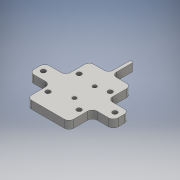
# Autodesk Inventor part: vertical carriage vasi
Saved by Autodesk Inventor 2016 SP1 (Build 200210100, 210)
## iProperties
Created: 2016-03-21
Part Number: vertical carriage vasi
Material: Generic
Document SubType Name: Modeling
Designer: ubik
Density: 1 g/cm^3
Appearance: Default
Author: ubik
Autodesk Inventor part; units mm, degrees
ref_plane "YZ Plane" through (0, 0, 0) normal (1, 0, 0) x (0, 1, 0)
ref_plane "XZ Plane" through (0, 0, 0) normal (0, 1, 0) x (-1, 0, 0)
ref_plane "XY Plane" through (0, 0, 0) normal (0, 0, 1) x (1, 0, 0)
sketch "Sketch1" plane through (0, 0, 0) normal (0, 0, 1) x (1, 0, 0)
  circle A0 centre (-10, 0) radius 1.5
  circle A1 centre (10, 0) radius 1.5
  circle A2 centre (-10, -20) radius 1.5
  circle A3 centre (10, -20) radius 1.5
  line L0 (-15, 10) -> (15, 10)
  line L1 (15, 10) -> (15, -30)
  line L2 (15, -30) -> (-15, -30)
  line L3 (-15, -30) -> (-15, 10)
  point P0 (0, 0)
  dimension "d0" = 3
  dimension "d1" = 3
  dimension "d2" = 20
  dimension "d3" = 10
  dimension "d4" = 3
  dimension "d5" = 3
  dimension "d6" = 20
  dimension "d7" = 20
  dimension "d8" = 20
  dimension "d9" = 10
  dimension "d10" = 30
  dimension "d11" = 15
  dimension "d12" = 40
  dimension "d13" = 10
  constraints: 8 end point, 4 centre point, 2 parallel, 1 horizontal, 1 perpendicular
  measures "d0" diameter of A0
  measures "d1" diameter of A1
  measures "d2" distance of A1.centre A0.centre
  measures "d3" distance of point (0, 0) A0.centre
  measures "d4" diameter of A2
  measures "d5" diameter of A3
  measures "d6" distance of A2.centre A0.centre
  measures "d7" distance of A3.centre A1.centre
  measures "d8" distance of A3.centre A2.centre
  measures "d9" horizontal distance of point (0, 0) A2.centre
  measures "d10" distance of L0.start L0.end
  measures "d11" distance from line of point (0, 0) L3
  measures "d12" distance of L2.end L0.start
  measures "d13" distance from line of point (0, 0) L0
extrude "Extrusion1" add sketch "Sketch1" along normal blind 5
sketch "Sketch2" plane through (0, 0, 5) normal (0, 0, 1) x (1, 0, 0)
  line L0 (0, 15.442053) -> (0, -37.541934) construction
  line L1 (-4, 15.442053) -> (-4, -37.541934) construction
  line L2 (-15, -30) -> (15, -30) construction
  line L3 (15, 10) -> (-15, 10)
  line L4 (15, -30) -> (15, 10)
  line L5 (7, 10) -> (7, -30)
  line L6 (7, 10) -> (15, 10)
  line L7 (7, -30) -> (15, -30)
  line L8 (6.3, 15.442053) -> (6.3, 10) construction
  line L9 (6.3, -30) -> (6.3, -37.541934) construction
  line L10 (-15, 10) -> (-15, -30)
  line L11 (15, -30) -> (15, 10)
  point P0 (0, 0)
  dimension "d16" = 4
  dimension "d96" = 0
  dimension "d97" = 0
  dimension "d141" = 22
  dimension "d152" = 0
  constraints: 16 end point, 4 vertical, 2 perpendicular, 2 point on line, 1 parallel
  measures "d16" distance between parallel lines of L0 L1
  measures "d96" distance between parallel lines of L3 L6
  measures "d97" distance between parallel lines of L2 L7
  measures "d141" distance between parallel lines of L5 L10
  measures "d152" distance between parallel lines of L11 L4
extrude "Extrusion2" add sketch "Sketch2" along normal blind 10
sketch "Sketch4" plane through (0, 0, 15) normal (0, 0, 1) x (1, 0, 0)
  circle A0 centre (10, 0) radius 3.25
  circle A1 centre (10, -20) radius 1.5 projected
  circle A2 centre (10, -20) radius 3.25
  point P0 (0, 0)
  point P1 (8.5, 0)
  point P2 (8.5, -20)
  dimension "d37" = 6.5
  dimension "d38" = 6.5
  constraints: 2 centre point, 2 coincident, 1 horizontal alignment
  measures "d37" diameter of A0
  measures "d38" diameter of A2
extrude "Extrusion3" [suppressed]
sketch "Sketch5" plane through (0, 0, 5) normal (0, 0, 1) x (1, 0, 0)
  line L0 (-4, 15.442053) -> (-4, -37.541934) construction
  line L1 (15, -30) -> (-15, -30)
  line L2 (7, 10) -> (-15, 10)
  line L3 (-3.3, 10) -> (1, 10)
  line L4 (4.5, -30) -> (-3.3, -30)
  line L5 (-3.3, -30) -> (-3.3, 10)
  line L6 (-2, 6) -> (1, 6)
  line L7 (4.5, -26) -> (-2, -26)
  line L8 (-2, -26) -> (-2, 6)
  line L9 (1, 10) -> (1, 6)
  line L10 (4.5, -26) -> (4.5, -30)
  line L11 (7, 10) -> (7, -30)
  point P0 (0, 0)
  point P1 (6.3, 10)
  point P2 (6.3, -30)
  point P3 (15, 10)
  dimension "d111" = 0.7
  dimension "d112" = 4
  dimension "d115" = 4
  dimension "d116" = 1.3
  dimension "d117" = 6
  dimension "d118" = 2.5
  dimension "d139" = 0
  dimension "d140" = 0
  constraints: 16 end point, 4 parallel, 2 horizontal, 2 perpendicular
  measures "d111" distance between parallel lines of L5 L0
  measures "d112" distance between parallel lines of L6 L3
  measures "d115" distance between parallel lines of L4 L7
  measures "d116" distance between parallel lines of L5 L8
  measures "d117" distance between parallel lines of L11 L9
  measures "d118" distance between parallel lines of L11 L10
  measures "d139" distance between parallel lines of L1 L4
  measures "d140" distance between parallel lines of L2 L3
extrude "Extrusion4" add sketch "Sketch5" along normal up to surface (10 mm away) contours L1 L5 L2 L9 L6 L8 L7 L10
sketch "Sketch8" plane through (0, 0, 0) normal (0, 0, -1) x (-1, 0, 0)
  line L0 (27, -15) -> (-27, -15)
  line L1 (-27, -15) -> (-27, -5)
  line L2 (-27, -5) -> (27, -5)
  line L3 (27, -5) -> (27, -15)
  line L4 (15, 10) -> (-15, 10) projected
  line L5 (-15, -30) -> (15, -30) projected
  circle A0 centre (23, -10) radius 1.5
  circle A1 centre (-23, -10) radius 1.5
  point P0 (0, 0)
  dimension "d77" = 10
  dimension "d78" = 40
  dimension "d79" = 15
  dimension "d80" = 3
  dimension "d81" = 3
  dimension "d82" = 46
  dimension "d83" = 54
  dimension "d84" = 23
  dimension "d85" = 27
  constraints: 8 end point, 2 centre point, 2 parallel, 1 horizontal, 1 perpendicular
  measures "d77" distance between parallel lines of L2 L0
  measures "d78" distance between parallel lines of L4 L5
  measures "d79" distance between parallel lines of L5 L0
  measures "d80" diameter of A0
  measures "d81" diameter of A1
  measures "d82" distance of A1.centre A0.centre
  measures "d83" distance of L1.end L2.end
  measures "d84" horizontal distance of point (0, 0) A0.centre
  measures "d85" distance from line of point (0, 0) L3
extrude "Extrusion5" add sketch "Sketch8" against normal up to surface (5 mm away)
sketch "Sketch3" plane through (0, 0, 5) normal (0, 0, 1) x (1, 0, 0)
  circle A0 centre (2, -2) radius 1.25
  circle A1 centre (2, -15) radius 1.25
  line L0 (-15, -30) -> (15, -30) projected
  line L1 (15, 10) -> (-15, 10) projected
  point P0 (0, 0)
  point P1 (7, -30)
  point P2 (6.3, 10)
  dimension "d23" = 2.5
  dimension "d24" = 2.5
  dimension "d25" = 15
  dimension "d26" = 2
  dimension "d27" = 2
  dimension "d28" = 12
  constraints: 2 centre point
  measures "d23" diameter of A0
  measures "d24" diameter of A1
  measures "d25" distance from line of L0 A1.centre
  measures "d26" horizontal distance of point (0, 0) A1.centre
  measures "d27" horizontal distance of point (0, 0) A0.centre
  measures "d28" distance from line of L1 A0.centre
hole "Hole1" at (2, -2, 5) at (2, -15, 5) direction (0, 0, -1) diameter 2.5 end through all
fillet "Fillet5" [suppressed]
fillet "Fillet7" [suppressed]
sketch "Sketch11" plane through (0, 0, 0) normal (0, 0, -1) x (-1, 0, 0)
  line L0 (15, -15) -> (13.5, -15)
  line L1 (13.5, -5) -> (15, -5)
  line L2 (-15, -5) -> (-13.5, -5)
  line L3 (-13.5, -15) -> (-15, -15)
  line L4 (15, -30) -> (15, -15)
  line L5 (-15, -15) -> (-15, -30)
  line L6 (-15, 10) -> (-15, -5)
  line L7 (15, -5) -> (15, 10)
  line L8 (-15, -30) -> (-13.5, -30)
  line L9 (13.5, -30) -> (15, -30)
  line L10 (-13.5, -30) -> (-13.5, -15)
  line L11 (-13.5, -5) -> (-13.5, 10)
  line L12 (13.5, 10) -> (13.5, -5)
  line L13 (13.5, -15) -> (13.5, -30)
  line L14 (15, 10) -> (13.5, 10)
  line L15 (-15, 10) -> (15, 10) projected
  line L16 (-15, 10) -> (-13.5, 10)
  point P0 (0, 0)
  dimension "d121" = 27
  constraints: 32 end point, 4 parallel, 2 collinear
  measures "d121" distance of L11.end L12.start
extrude "Extrusion7" cut sketch "Sketch11" against normal through all
fillet "Fillet9" radius 3 12 edges at (-27, -15, 2.5) (-13.5, -30, 2.5) (13.5, -30, 7.5) (-27, -5, 2.5) (-13.5, -5, 2.5) (-13.5, 10, 2.5) (13.5, -15, 7.5) (27, -15, 2.5) (27, -5, 2.5) (13.5, -5, 7.5) (13.5, 10, 7.5) (-13.5, -15, 2.5)
sketch "Sketch12" plane through (4, -30, 4) normal (0, -1, 0) x (1, 0, 0)
  line L0 (0.5, 11) -> (-7.3, 11) projected
  circle A0 centre (-2, 3) radius 1.5
  line L1 (0.5, 1) -> (3, 1) projected
  line L2 (6.5, -4) -> (-14.5, -4) projected
  line L3 (6.5, 11) -> (6.5, -4) projected
  line L4 (-14.5, -4) -> (-14.5, 1) projected
  line L5 (-7.3, 1) -> (-7.3, 11) projected
  line L6 (-14.5, 1) -> (-7.3, 1) projected
  line L7 (3, 11) -> (6.5, 11) projected
  line L8 (3, 1) -> (3, 11) projected
  line L9 (0.5, 1) -> (0.5, 11) projected
  point P0 (-4, -4)
  dimension "d126" = 3
  dimension "d129" = 3
  constraints: 1 centre point
  measures "d126" diameter of A0
extrude "Extrusion8" [suppressed]
sketch "Sketch14" plane through (0, 0, 0) normal (0, 0, -1) x (-1, 0, 0)
  line L0 (10.5, 10) -> (-10.5, 10) projected
  line L1 (-1, 10) -> (1, 10)
  line L2 (1, 10) -> (1, 24)
  line L3 (1, 24) -> (-1, 24)
  line L4 (-1, 24) -> (-1, 10)
  point P0 (0, 0)
  dimension "d142" = 14
  dimension "d143" = 1
  dimension "d144" = 1
  constraints: 8 end point, 2 parallel, 1 horizontal, 1 perpendicular, 1 point on line
  measures "d142" distance of L1.end L2.end
  measures "d143" distance from line of point (0, 0) L4
  measures "d144" distance from line of point (0, 0) L2
extrude "Extrusion10" add sketch "Sketch14" against normal up to surface (15 mm away)
fillet "Fillet10" radius 3 2 edges at (-1, 10, 7.5) (1, 10, 2.5)
fillet "Fillet11" radius 1 2 edges at (-1, 24, 7.5) (1, 24, 7.5)
sketch "Sketch15" plane through (-3.3, -30, 15) normal (0, 0, 1) x (1, 0, 0)
  arc A0 (2.3, 53) -> (4.3, 53) centre (3.3, 53) ccw
  line L0 (2.3, 43) -> (2.3, 53)
  arc A1 (0, 40.08281) -> (2.3, 43) centre (-0.7, 43) ccw
  line L1 (0, 0) -> (0, 36)
  line L2 (7.8, 0) -> (0, 0)
  line L3 (7.8, 4) -> (7.8, 0)
  line L4 (1.3, 4) -> (7.8, 4)
  line L5 (1.3, 36) -> (1.3, 4)
  line L6 (4.3, 36) -> (1.3, 36)
  line L7 (4.3, 53) -> (4.3, 36)
  line L8 (7.3, 40) -> (7.8, 40)
  arc A2 (4.3, 43) -> (6.8, 40.04196) centre (7.3, 43) ccw
  line L9 (4.3, 53) -> (4.3, 36)
  line L10 (1.3, 36) -> (1.3, 4)
  line L11 (1.3, 36) -> (0, 36)
  line L12 (0, 0) -> (0, 36)
  point P0 (3.3, 30)
  constraints: 8 end point, 4 centre point, 2 point on circle, 1 perpendicular, 1 other
extrude "Extrusion11" cut sketch "Sketch15" against normal up to surface (10 mm away)
sketch "Sketch16" plane through (10, 0, 5) normal (0, 0, -1) x (-1, 0, 0)
  circle A0 centre (0, 0) radius 1.5 projected
  circle A1 centre (0, -20) radius 1.5 projected
  point P0 (10, 0)
extrude "Extrusion12" cut sketch "Sketch16" against normal through all
sketch "Sketch17" plane through (-3.3, 6, 15) normal (0, 0, 1) x (1, 0, 0)
  line L0 (4.3, 0) -> (0, 0)
  line L1 (4.3, 17) -> (4.3, 0)
  arc A0 (4.3, 17) -> (2.3, 17) centre (3.3, 17) ccw
  line L2 (2.3, 7) -> (2.3, 17)
  arc A1 (0, 4.08281) -> (2.3, 7) centre (-0.7, 7) ccw
  line L3 (0, 0) -> (0, 4.08281)
  point P0 (3.3, -6)
sketch "Sketch17 outline for Extrusion13" plane through (-3.3, 6, 15) normal (0, 0, 1) x (1, 0, 0)
  line L0 (0, 4.08281) -> (0, 0)
  arc A0 (2.3, 7) -> (0, 4.08281) centre (-0.7, 7) cw
  line L1 (2.3, 17) -> (2.3, 7)
  arc A1 (4.3, 17) -> (2.3, 17) centre (3.3, 17) ccw
  line L2 (4.3, 0) -> (4.3, 17)
  line L3 (0, 0) -> (4.3, 0)
extrude "Extrusion13" cut sketch "Sketch17 outline for Extrusion13" against normal up to surface (10 mm away)
sketch "Sketch18" plane through (0, 0, 15) normal (0, 0, 1) x (1, 0, 0)
  circle A0 centre (10, 0) radius 1.5
  circle A1 centre (10, -20) radius 1.5
  arc A2 (13.5, 7) -> (10.5, 10) centre (10.5, 7) ccw
  line L0 (10.5, 10) -> (7, 10)
  line L1 (7, 10) -> (7, -30)
  line L2 (7, -30) -> (10.5, -30)
  arc A3 (10.5, -30) -> (13.5, -27) centre (10.5, -27) ccw
  line L3 (13.5, -27) -> (13.5, -18)
  arc A4 (15, -15.401924) -> (13.5, -18) centre (16.5, -18) ccw
  line L4 (15, -4.598076) -> (15, -15.401924)
  arc A5 (13.5, -2) -> (15, -4.598076) centre (16.5, -2) ccw
  line L5 (13.5, -2) -> (13.5, 7)
  point P0 (0, 0)
extrude "Extrusion14" cut sketch "Sketch18" against normal up to surface (10 mm away)
sketch "Sketch13" plane through (-10.5, -30, 0) normal (0, -1, 0) x (1, 0, 0)
  line L0 (21, 4) -> (21, 0) projected
  line L1 (0, 0) -> (0, 4) projected
  line L2 (21, 0) -> (0, 0) projected
  circle A0 centre (11, 8) radius 1.5
  line L3 (19.5, 4) -> (21, 4) projected
  line L4 (19.5, 4) -> (19.5, 14) projected
  line L5 (17.5, 14) -> (19.5, 14) projected
  line L6 (17.5, 4) -> (17.5, 14) projected
  line L7 (15, 4) -> (17.5, 4) projected
  line L8 (15, 4) -> (15, 14) projected
  line L9 (15, 14) -> (7.2, 14) projected
  line L10 (7.2, 4) -> (7.2, 14) projected
  line L11 (0, 4) -> (7.2, 4) projected
  point P0 (10.5, 0)
  dimension "d132" = 3
  dimension "d133" = 21
  dimension "d134" = 4
  dimension "d136" = 11
  dimension "d149" = 8
  constraints: 1 centre point
  measures "d132" diameter of A0
  measures "d133" distance of L1.end L0.start
  measures "d134" distance of L1.start L1.end
  measures "d136" distance from line of L1 A0.centre
  measures "d149" distance from line of L2 A0.centre
sketch "Sketch9" plane through (0, 0, 5) normal (0, 0, 1) x (1, 0, 0)
  circle A0 centre (-10, 0) radius 1.5 projected
  circle A1 centre (2, -2) radius 1.25 projected
  circle A2 centre (10, 0) radius 1.5 projected
  circle A3 centre (23, -10) radius 1.5 projected
  circle A4 centre (10, -20) radius 1.5 projected
  circle A5 centre (2, -15) radius 1.25 projected
  circle A6 centre (-10, -20) radius 1.5 projected
  circle A7 centre (-23, -10) radius 1.5 projected
  point P0 (0, 0)
equation "\"d3\" = 0.5 * d2"
equation "\"d7\" = d6"
equation "\"d8\" = d2"
equation "\"d9\" = d3"
equation "\"d11\" = 0.5 * d10"
equation "\"d13\" = -0.5 * d6 + 0.5 * d12"
equation "\"d37\" = d38"
equation "\"d115\" = d112"
equation "\"d79\" = -0.5 * d77 + 0.5 * d78"
equation "\"d84\" = 0.5 * d82"
equation "\"d85\" = 0.5 * d83"
equation "\"d27\" = d26"
body "Solid1"
